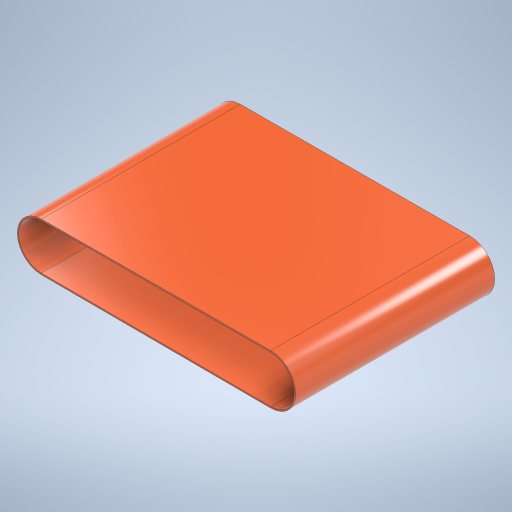
# Autodesk Inventor part: faja
Saved by Autodesk Inventor 2023 (Build 270158030, 158C)
## iProperties
Created: 2022-05-25
Part Number: faja
Material: Genérico
Document SubType Name: Modeling
Designer: isaac
Density: 1 g/cm^3
Appearance: Valor por defecto
Author: isaac
Autodesk Inventor part; units mm, degrees
ref_plane "YZ Plane" through (0, 0, 0) normal (1, 0, 0) x (0, 1, 0)
ref_plane "XZ Plane" through (0, 0, 0) normal (0, 1, 0) x (-1, 0, 0)
ref_plane "XY Plane" through (0, 0, 0) normal (0, 0, 1) x (1, 0, 0)
sketch "Boceto1" plane through (0, 0, 0) normal (0, 0, 1) x (1, 0, 0)
  arc A0 (-750.5267, 157.9991) -> (-750.5267, -157.9991) centre (-750, 0) ccw
  arc A1 (749.4567, -162.9991) -> (749.4567, 162.9991) centre (750, 0) ccw
  line L0 (-750.5267, 157.9991) -> (749.4567, 162.9991)
  line L1 (749.4567, -162.9991) -> (-750.5267, -157.9991)
  line L2 (749.49, 152.9991) -> (-750.4933, 147.9992)
  arc A2 (-750.4933, 147.9992) -> (-750.4933, -147.9992) centre (-750, 0) ccw
  line L3 (-750.4933, -147.9992) -> (749.49, -152.9991)
  arc A3 (749.49, -152.9991) -> (749.49, 152.9991) centre (750, 0) ccw
  point P0 (0, 0)
  dimension "d0" = 1500
  dimension "d1" = 326
  dimension "d2" = 316
  dimension "d3" = 750
  dimension "d4" = 10
  constraints: 8 end point, 8 point on circle, 4 centre point, 4 tangent, 2 horizontal alignment, 3 other
  measures "d0" distance of A1.centre A0.centre
  measures "d1" diameter of A1
  measures "d2" diameter of A0
  measures "d3" distance of point (0, 0) A0.centre
  measures "d4" radial gap between concentric circles of A1 A3
extrude "Extrusión1" add sketch "Boceto1" along normal blind 1300
equation "\"d3\" = 0.5 * d0"
